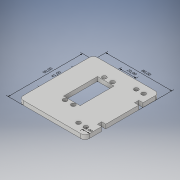
# Autodesk Inventor part: Ground
Saved by Autodesk Inventor 2019 (Build 230136000, 136)
## iProperties
Created: 2018-06-10
Part Number: Ground
Material: Ogólny
Document SubType Name: Modeling
Designer: Kamil
Density: 1 g/cm^3
Appearance: Domyślna
Author: Kamil
Autodesk Inventor part; units mm, degrees
ref_plane "YZ Plane" through (0, 0, 0) normal (1, 0, 0) x (0, 1, 0)
ref_plane "XZ Plane" through (0, 0, 0) normal (0, 1, 0) x (-1, 0, 0)
ref_plane "XY Plane" through (0, 0, 0) normal (0, 0, 1) x (1, 0, 0)
sketch "Szkic1" plane through (0, 0, 0) normal (0, 1, 0) x (-1, 0, 0)
  line L0 (-35, 45) -> (35, 45)
  line L1 (40, 40) -> (40, -40)
  line L2 (35, -45) -> (-35, -45)
  line L3 (-40, -40) -> (-40, -25)
  line L4 (-40, 45) -> (40, -45) construction
  line L5 (40, 45) -> (-40, -45) construction
  arc A0 (40, 40) -> (35, 45) centre (35, 40) ccw
  arc A1 (-35, 45) -> (-40, 40) centre (-35, 40) ccw
  arc A2 (-40, -40) -> (-35, -45) centre (-35, -40) ccw
  arc A3 (35, -45) -> (40, -40) centre (35, -40) ccw
  line L6 (15, -25) -> (-5, -25)
  line L7 (-5, -25) -> (-5, 16)
  line L8 (-5, 16) -> (15, 16)
  line L9 (15, 16) -> (15, -25)
  circle A4 centre (10, 19.25) radius 2.5
  circle A5 centre (0, 19.25) radius 2.5
  circle A6 centre (10, -28.25) radius 2.5
  circle A7 centre (0, -28.25) radius 2.5
  line L10 (-40, 25) -> (-35, 25)
  line L11 (-35, 25) -> (-35, 20)
  line L12 (-35, 20) -> (-40, 20)
  line L13 (-40, -20) -> (-35, -20)
  line L14 (-35, -20) -> (-35, -25)
  line L15 (-35, -25) -> (-40, -25)
  line L16 (-40, 20) -> (-40, 25)
  line L17 (-40, 25) -> (-40, 40)
  line L18 (-40, -20) -> (-40, 20)
  circle A8 centre (-22, -35) radius 2.5
  circle A9 centre (-22, 35) radius 2.5
  circle A10 centre (-31, 35) radius 2.5
  circle A11 centre (-31, -35) radius 2.5
  point P0 (0, 0)
  dimension "d0" = 80
  dimension "d1" = 90
  dimension "d2" = 5
  dimension "d3" = 20
  dimension "d4" = 41
  dimension "d5" = 5
  dimension "d6" = 5
  dimension "d7" = 5
  dimension "d8" = 5
  dimension "d18" = 5
  dimension "d19" = 5
  dimension "d20" = 5
  dimension "d21" = 5
  dimension "d50" = 5
  dimension "d52" = 5
  dimension "d53" = 5
  dimension "d54" = 5
  constraints: 38 end point, 14 tangent, 12 centre point, 9 parallel, 9 point on line, 8 point on circle, 4 horizontal, 4 perpendicular, 3 equal radius, 2 midpoint
  measures "d0" distance of L4.end L5.end
  measures "d1" distance of L5.start L4.end
  measures "d2" radius of A0
  measures "d3" distance of L7.end L8.end
  measures "d4" distance of L6.end L7.end
  measures "d5" diameter of A4
  measures "d6" diameter of A5
  measures "d7" diameter of A6
  measures "d8" diameter of A7
  measures "d18" distance of L11.end L12.end
  measures "d19" distance of L10.end L11.end
  measures "d20" distance of L14.end L3.end
  measures "d21" distance of L13.end L14.end
  measures "d50" diameter of A8
  measures "d52" diameter of A9
  measures "d53" diameter of A10
  measures "d54" diameter of A11
extrude "Wyciągnięcie proste3" add sketch "Szkic1" along normal blind 5 contours L0 A0 L1 A3 L2 A2 L3 L15 L14 L13 L18 L12 L11 L10 L17 A1
